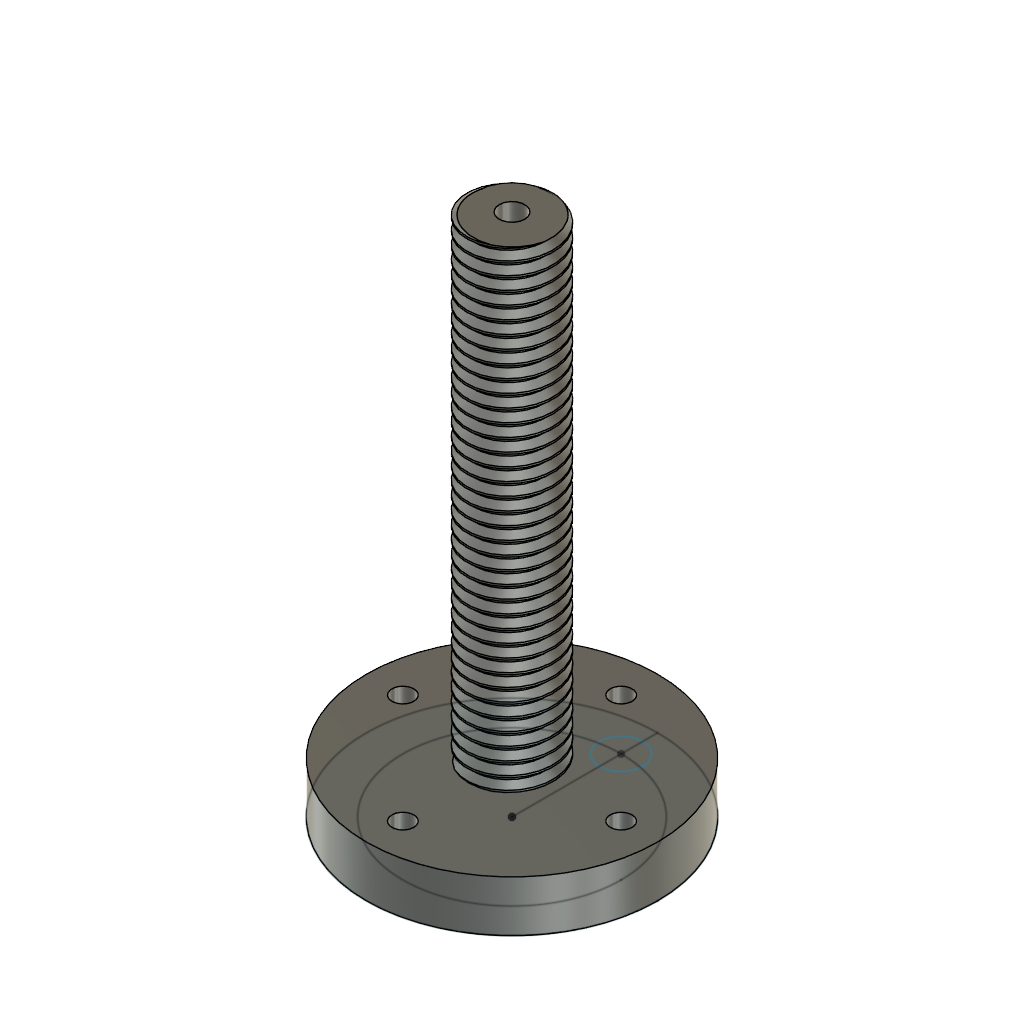
Pastaka_kinnitus_robotile (Autodesk Fusion 360 design; units mm, degrees)
part number: 2026-09-11-19-18-27-527
Autodesk Fusion 360 part; units mm, degrees
note: some values were not read from the file. Set by a fixed rule: which sketch regions a step uses; the direction of a hole.
sketch "Sketch1" plane through (0, 0, 0) normal (0, 0, 1) x (1, 0, 0)
  circle A0 centre (0, 0) radius 20
  line L0 (0, 0) -> (0, 20)
  circle A1 centre (0, 0) radius 15
  circle A2 centre (0, 15) radius 2.9703
  dimension "d1" = 40
  dimension "d2" = 30
  constraint coincident A0.centre L0.start
  constraint coincident A0 L0.end
  constraint vertical L0
  constraint coincident A1 A2.centre
  constraint coincident L0 A2.centre
  measures "d1" diameter of A0
  measures "d2" diameter of A1
extrude "Extrude1" add sketch "Sketch1" along normal blind 7 contours A0 | L0 A1 A2 | A1 A2 | L0 A1 A2 | L0 A1 A2 | L0 A1 A2
hole "Hole1" at (0, 15, 0) direction (0, 0, 1) diameter 3 depth 7 tip angle 118
pattern_circular "C-Pattern1" count 4 over 360 about axis through (0, 0, 1.75) along (0, 0, 1) of "Hole1"
sketch "Sketch2" plane through (0, 0, 7) normal (0, 0, 1) x (-1, 0, 0)
  circle A0 centre (-15, 0) radius 1.5
  circle A1 centre (0, 15) radius 1.5
  circle A2 centre (15, 0) radius 1.5
  circle A3 centre (0, -15) radius 1.5
  circle A4 centre (0, 0) radius 20
  circle A5 centre (0, 0) radius 6
  dimension "d10" = 12
  constraint coincident A4.centre A5.centre
  measures "d10" diameter of A5
extrude "Extrude2" add sketch "Sketch2" along normal blind 65 contours A5
thread "Thread1" "ISO Metric profile 12.0 M12x1.75 M12x1.75 6g" major diameter 11.8335 minor diameter 9.8365 pitch 1.75 angle 60 modelled right hand crest width 0.2518 on face at (-5.9702, 0.5974, 28.6667) crest through (-5.9168, 0, 6.5625)
sketch "Sketch3" plane through (0, 0, 72) normal (0, 0, 1) x (-1, 0, 0)
  circle A0 centre (0, 0) radius 1.75
  spline S0 degree 3 poles (4.9113, -0.2623) (5.009, 0.3795) (4.9782, 1.0342) (4.6661, 2.3201) (4.3788, 2.9365) (3.5734, 4.047) (3.0556, 4.525) (1.8475, 5.2724) (1.164, 5.5268) (-0.046, 5.7279) (-0.552, 5.7436) (-1.5659, 5.6421) (-2.0691, 5.5224) (-2.5504, 5.3388) knots 0 0 0 0 0.194743 0.194743 0.396632 0.396632 0.605663 0.605663 0.821834 0.821834 0.972548 0.972548 1.12654 1.12654 1.12654 1.12654
  arc A1 (-2.5504, 5.3388) -> (-5.7725, 1.2985) centre (0, 0) ccw
  spline S1 degree 3 poles (-5.7725, 1.2985) (-5.878, 0.5497) (-5.8384, -0.2123) (-5.471, -1.6538) (-5.1556, -2.3215) (-4.2974, -3.4763) (-3.7702, -3.9577) (-2.5795, -4.6749) (-1.9322, -4.9117) (-0.8145, -5.0837) (-0.3645, -5.0937) (0.5155, -4.9952) (0.9418, -4.8901) (1.3486, -4.7298) knots 0 0 0 0 0.226861 0.226861 0.446562 0.446562 0.659101 0.659101 0.864475 0.864475 0.999343 0.999343 1.130941 1.130941 1.130941 1.130941
  arc A2 (1.3486, -4.7298) -> (4.9113, -0.2623) centre (0, 0) ccw
  dimension "d15" = 3.5
  constraint coincident A0.centre A1.centre
  measures "d15" diameter of A0
extrude "Extrude3" cut sketch "Sketch3" against normal blind 65 contours A0
